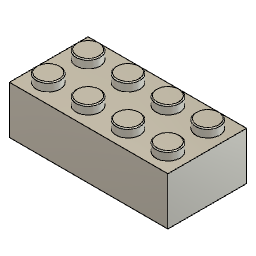
Day1LegoBrickUpdated v2 (Autodesk Fusion 360 design; units mm, degrees)
Autodesk Fusion 360 part; units mm, degrees
sketch "Sketch1" plane through (0, 0, 0) normal (0, 1, 0) x (1, 0, 0) in component "Brick"
  line L0 (0, 0) -> (31.8, 0)
  line L1 (31.8, 0) -> (31.8, 15.8)
  line L2 (31.8, 15.8) -> (0, 15.8)
  line L3 (0, 15.8) -> (0, 0)
  dimension "d1" = 31.8
  dimension "d2" = 15.8
  constraint horizontal L0
  constraint vertical L1
  constraint horizontal L2
  constraint vertical L3
  constraint coincident L0.start L3.end
  measures "d1" distance of L0.start L0.end
  measures "d2" distance of L0.start L2.end
extrude "Extrude1" add sketch "Sketch1" along normal blind 9.6 in component "Brick"
sketch "Sketch2" plane through (0, 9.6, 0) normal (0, 1, 0) x (-1, 0, 0) in component "Brick"
  line L0 (0, -15.8) -> (0, 0)
  line L1 (0, 0) -> (-31.8, 0)
  line L2 (-31.8, 0) -> (-31.8, -15.8)
  circle A0 centre (-3.9, -11.9) radius 2.4
  line L3 (-31.8, -15.8) -> (0, -15.8)
  dimension "d5" = 4.8
  dimension "d6" = 3.9
  dimension "d7" = 3.9
  measures "d5" diameter of A0
  measures "d6" distance of A0.centre L3
  measures "d7" distance of L0 A0.centre
extrude "Extrude2" add sketch "Sketch2" along normal blind 1.7 contours A0 in component "Brick"
pattern_linear "R-Pattern1" count 4 spacing 8 along (1, 0, 0) count 2 spacing 8 along (0, 0, 1) of "Extrude2" in component "Brick"
shell "Shell1" thickness 1.2 removed faces 1 at (21.2, 0, -5.2667) in component "Brick"
sketch "Sketch3" plane through (0, 8.4, 0) normal (0, -1, 0) x (1, 0, 0) in component "Brick"
  circle A0 centre (27.9, -3.9) radius 1.2
  circle A1 centre (19.9, -3.9) radius 1.2
  circle A2 centre (11.9, -3.9) radius 1.2
  circle A3 centre (3.9, -3.9) radius 1.2
  circle A4 centre (27.9, -11.9) radius 1.2
  circle A5 centre (19.9, -11.9) radius 1.2
  circle A6 centre (11.9, -11.9) radius 1.2
  circle A7 centre (3.9, -11.9) radius 1.2
  line L0 (1.2, -1.2) -> (1.2, -14.6)
  line L1 (1.2, -14.6) -> (30.6, -14.6)
  line L2 (30.6, -14.6) -> (30.6, -1.2)
  line L3 (30.6, -1.2) -> (1.2, -1.2)
  line L4 (19.9, -11.9) -> (27.9, -3.9) construction
  circle A8 centre (23.9, -7.9) radius 3.255
  circle A9 centre (23.9, -7.9) radius 2.395
  dimension "d15" = 6.51
  dimension "d16" = -0.86
  constraint coincident A5.centre L4.start
  constraint coincident A0.centre L4.end
  constraint midpoint L4 A8.centre
  measures "d15" diameter of A8
extrude "Extrude3" add sketch "Sketch3" along normal blind 8.1 contours A8 in component "Brick"
pattern_linear "R-Pattern2" count 3 spacing 8 along (-1, 0, 0) of "Extrude3" in component "Brick"
fillet "Fillet1" radius 0.2 8 edges at (30.1376, 11.3, -4.7679) (30.1376, 11.3, -12.7679) (22.1376, 11.3, -4.7679) (22.1376, 11.3, -12.7679) (14.1376, 11.3, -4.7679) (6.1376, 11.3, -4.7679) (6.1376, 11.3, -12.7679) (14.1376, 11.3, -12.7679) in component "Brick"
component "Brick" placed x (1, 0, 0) y (0, 1, 0) z (0, 0, 1) at (0, 0, 0)
